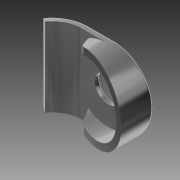
# Autodesk Inventor part: Pieza4
Saved by Autodesk Inventor 2013 (Build 170138000, 138)
## iProperties
Created: 2013-06-05
Part Number: Pieza4
Material: Acero
Document SubType Name: Modeling
Designer: BRAYAN
Density: 1 g/cm^3
Author: BRAYAN
Autodesk Inventor part; units mm, degrees
ref_plane "XZ Plane" through (0, 0, 0) normal (0, 1, 0) x (-1, 0, 0)
ref_plane "XY Plane" through (0, 0, 0) normal (0, 0, 1) x (1, 0, 0)
sketch "Boceto1" plane through (0, 0, 0) normal (0, 0, 1) x (1, 0, 0)
  line L0 (2, 7.1352) -> (2, -10.5453)
  line L1 (14, 1) -> (14, -9)
  line L2 (14, -9) -> (12, -9)
  line L3 (12, -9) -> (12, -1)
  line L4 (14, 1) -> (8, 1)
  line L5 (8, 1) -> (8, 0.8)
  line L6 (8, 0.8) -> (6, 0.8)
  line L7 (6, 0.8) -> (6, -1)
  line L8 (6, -1) -> (12, -1)
  line L9 (6, 0) -> (2, 0)
  point P0 (0, 0)
  point P1 (14, -0.5)
  dimension "d63" = 2
  dimension "d64" = 10
  dimension "d65" = 6
  dimension "d66" = 0.2
  dimension "d67" = 2
  dimension "d68" = 1.8
  dimension "d69" = 6
  dimension "d70" = 8
  dimension "d72" = 4
  constraints: 20 end point, 5 perpendicular, 2 point on line, 1 parallel
  measures "d63" distance of L1.end L2.end
  measures "d64" distance of L1.start L1.end
  measures "d65" distance of L1.start L4.end
  measures "d66" distance of L4.end L5.end
  measures "d67" distance of L5.end L6.end
  measures "d68" distance of L6.end L7.end
  measures "d69" distance of L7.end L3.end
  measures "d70" distance of L2.end L3.end
  measures "d72" distance of L9.start L9.end
revolve "Revolución3" add sketch "Boceto1" angle 360 about axis through (2, 7.1352, 0) along (0, -1, 0)
sketch "Boceto5" plane through (0, 0, 0) normal (0, 0, 1) x (1, 0, 0)
  line L0 (-0.0004, -1) -> (1.9996, -1)
  line L1 (-0.0004, -1) -> (-4.0004, -1)
  line L2 (-0.0004, -1) -> (3.9996, -1) construction
  line L3 (-4.0004, -1) -> (-6.0004, -1)
  line L4 (-6.0004, -1) -> (-6.0004, -10)
  arc A0 (-6.0004, -1) -> (-13.364, -4.8254) centre (-6.0004, -10) ccw
  arc A1 (-6.0004, 1) -> (-15.0004, -3.6754) centre (-6.0004, -10) ccw
  line L5 (-15.0004, -3.6754) -> (-13.364, -4.8254)
  line L6 (1.9996, 1) -> (-6.0004, 1)
  line L7 (1.9996, -1) -> (1.9996, 1)
  point P0 (0, 0)
  dimension "d106" = 180
  dimension "d107" = 2
  dimension "d108" = 4
  dimension "d110" = 2
  dimension "d111" = 9
  dimension "d112" = 22
  dimension "d114" = 2
  constraints: 16 end point, 4 point on circle, 2 centre point, 2 coincident, 2 collinear, 2 horizontal, 2 perpendicular, 1 tangent
  measures "d106" angle of L1 L2
  measures "d107" distance of L0.start L0.end
  measures "d108" distance of L0.start L1.end
  measures "d110" distance of L1.end L3.end
  measures "d111" distance of L3.end L4.end
  measures "d112" diameter of A1
  measures "d114" distance of L5.start L5.end
sketch "Boceto6" plane through (0, 0, 0) normal (0, 0, 1) x (1, 0, 0)
  line L0 (0, 0) -> (0, 1)
  line L1 (0, 1) -> (-4, 1)
  line L2 (-4, 1) -> (-4, -1)
  line L3 (0, 1) -> (14, 1)
  line L4 (14, 1) -> (14, -9)
  line L5 (-2, -5) -> (14, -9)
  line L6 (-2, -5) -> (-4, -1)
  line L7 (14, -9) -> (17.4985, -12.2615)
  line L8 (17.4985, -12.2615) -> (-11.8502, -17.8502)
  line L9 (-4, -1) -> (-12.2858, -1)
  line L10 (-12.2858, -1) -> (-11.8502, -17.8502)
  dimension "d97" = 1
  dimension "d98" = 4
  dimension "d99" = 2
  dimension "d100" = 14
  dimension "d101" = 10
  constraints: 22 end point, 4 perpendicular, 1 parallel, 1 vertical
  measures "d97" distance of L0.start L0.end
  measures "d98" distance of L0.end L1.end
  measures "d99" distance of L1.end L2.end
  measures "d100" distance of L0.end L3.end
  measures "d101" distance of L3.end L4.end
extrude "Extrusión4" cut sketch "Boceto6" along normal through all both and the other way through all contours L6 L5 L7 L8 L10 L9
extrude "Extrusión5" add sketch "Boceto5" along normal mid plane 24
delete faces "Suprimir cara4" heal yes whole lump no faces at (1.9996, 0.2, 1.3333)
delete faces "Suprimir cara5" heal yes whole lump no faces at (-9.9989, 0.7503, 0.1588)
fillet "Empalme8" radius 1 1 edges at (-2, 0.8, 0)
fillet "Empalme9" radius 2 2 edges at (-2, -5, 10.2394) (-2, -5, -10.2394)
fillet "Empalme10" radius 1 5 edges at (14, 1, 0) (-2.0004, 1, 12) (-11.0714, -0.2386, 12) (-2.0004, 1, -12) (-11.0714, -0.2386, -12)
sketch "Boceto7" plane through (0, 0, 12) normal (0, 0, 1) x (1, 0, 0)
  arc A0 (-6.0004, 0) -> (-14.1822, -4.2504) centre (-6.0004, -10) ccw projected
  line L0 (-14.1822, -4.2504) -> (-13.364, -4.8254) projected
  arc A1 (-6.0004, -1) -> (-13.364, -4.8254) centre (-6.0004, -10) ccw projected
  line L1 (-6.0004, -1) -> (1.9996, -1) projected
  line L2 (1.9996, 0) -> (1.9996, -1) projected
  line L3 (-6.0004, 0) -> (1.9996, 0) projected
  line L4 (-6.0004, -10) -> (-6.0004, 7.6016)
  line L5 (-6.0004, 7.6016) -> (-6.0004, -22.2322)
  point P0 (0, 0)
  constraints: 4 end point, 1 collinear, 1 perpendicular
sketch "Boceto8" plane through (0, 0, -12) normal (0, 0, -1) x (-1, 0, 0)
  arc A0 (14.1822, -4.2504) -> (6.0004, 0) centre (6.0004, -10) ccw projected
  line L0 (2.7958, 0) -> (6.0004, 0) projected
  line L1 (-1.9996, 0) -> (2.7958, 0) projected
  line L2 (-1.9996, 0) -> (-1.9996, -1) projected
  line L3 (-1.9996, -1) -> (6.0004, -1) projected
  arc A1 (13.364, -4.8254) -> (6.0004, -1) centre (6.0004, -10) ccw projected
  line L4 (13.364, -4.8254) -> (14.1822, -4.2504) projected
  line L5 (6.0004, -10) -> (6.0004, 7.6678)
  line L6 (6.0004, 7.6678) -> (6.0004, -22.166)
  point P0 (0, 0)
  constraints: 4 end point, 1 collinear, 1 perpendicular
ref_plane "Plano de trabajo2" through (2, 0, 0) normal (1, 0, 0) x (0, 1, 0)
